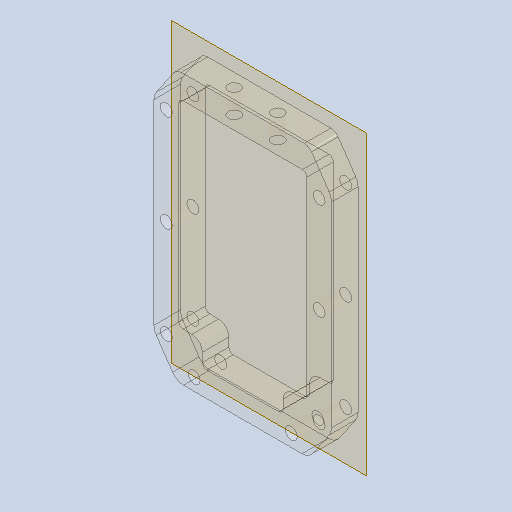
# Autodesk Inventor part: _inner
Saved by Autodesk Inventor 2024.3 (Build 283343000, 343)
## iProperties
Created: 2024-09-09
Part Number: _inner
Material: PMMA 플라스틱
Document SubType Name: Modeling
Designer: gretc
Density: 1.188 g/cm^3
Appearance: 폴리카보네이트 - 선명
Mass: 6.58685 g
Surface Area: 43.9029 cm^2
Volume: 5.54449 cm^3
Author: gretc
Autodesk Inventor part; units mm, degrees
ref_plane "YZ Plane" through (0, 0, 0) normal (1, 0, 0) x (0, 1, 0)
ref_plane "XZ Plane" through (0, 0, 0) normal (0, 1, 0) x (-1, 0, 0)
ref_plane "XY Plane" through (0, 0, 0) normal (0, 0, 1) x (1, 0, 0)
ref_plane "작업 평면1" through (0, 0, 0) normal (0, 0, 1) x (1, 0, 0)
sketch "스케치1" plane through (0, 0, 0) normal (0, 0, 1) x (1, 0, 0)
  arc A0 (-19.5808, 6.2636) -> (-20.1, 4.5766) centre (-17.1, 4.5766) ccw projected
  line L0 (-20.1, -39.6766) -> (-20.1, 4.5766) projected
  arc A1 (-20.1, -39.6766) -> (-19.5808, -41.3636) centre (-17.1, -39.6766) ccw projected
  line L1 (-15.8929, -46.7869) -> (-19.5808, -41.3636) projected
  arc A2 (-15.8929, -46.7869) -> (-13.4121, -48.1) centre (-13.4121, -45.1) ccw projected
  line L2 (13.4121, -48.1) -> (-13.4121, -48.1) projected
  arc A3 (13.4121, -48.1) -> (15.8929, -46.7869) centre (13.4121, -45.1) ccw projected
  line L3 (19.5808, -41.3636) -> (15.8929, -46.7869) projected
  arc A4 (19.5808, -41.3636) -> (20.1, -39.6766) centre (17.1, -39.6766) ccw projected
  line L4 (20.1, 4.5766) -> (20.1, -39.6766) projected
  arc A5 (20.1, 4.5766) -> (19.5808, 6.2636) centre (17.1, 4.5766) ccw projected
  line L5 (15.5953, 12.1246) -> (19.5808, 6.2636) projected
  arc A6 (15.5953, 12.1246) -> (13.9414, 13) centre (13.9414, 11) ccw projected
  line L6 (7.65, 13) -> (13.9414, 13) projected
  arc A7 (9.15, 11.5) -> (7.65, 13) centre (7.65, 11.5) ccw projected
  line L7 (9.15, 11.5) -> (9.15, 10) projected
  arc A8 (9.15, 10) -> (11.5, 7.65) centre (11.5, 10) ccw projected
  line L8 (11.5, 7.65) -> (13.5, 7.65) projected
  arc A9 (14.5, 6.65) -> (13.5, 7.65) centre (13.5, 6.65) ccw projected
  line L9 (14.5, 6.65) -> (14.5, -36.15) projected
  arc A10 (13.5, -37.15) -> (14.5, -36.15) centre (13.5, -36.15) ccw projected
  line L10 (13.5, -37.15) -> (11.5, -37.15) projected
  arc A11 (11.5, -37.15) -> (9.15, -39.5) centre (11.5, -39.5) ccw projected
  line L11 (9.15, -39.5) -> (9.15, -41.5) projected
  arc A12 (8.15, -42.5) -> (9.15, -41.5) centre (8.15, -41.5) ccw projected
  line L12 (8.15, -42.5) -> (-8.15, -42.5) projected
  arc A13 (-9.15, -41.5) -> (-8.15, -42.5) centre (-8.15, -41.5) ccw projected
  line L13 (-9.15, -41.5) -> (-9.15, -39.5) projected
  arc A14 (-9.15, -39.5) -> (-11.5, -37.15) centre (-11.5, -39.5) ccw projected
  line L14 (-11.5, -37.15) -> (-13.5, -37.15) projected
  arc A15 (-14.5, -36.15) -> (-13.5, -37.15) centre (-13.5, -36.15) ccw projected
  line L15 (-14.5, -36.15) -> (-14.5, 6.65) projected
  arc A16 (-13.5, 7.65) -> (-14.5, 6.65) centre (-13.5, 6.65) ccw projected
  line L16 (-13.5, 7.65) -> (-11.5, 7.65) projected
  arc A17 (-11.5, 7.65) -> (-9.15, 10) centre (-11.5, 10) ccw projected
  line L17 (-9.15, 10) -> (-9.15, 11.5) projected
  arc A18 (-7.65, 13) -> (-9.15, 11.5) centre (-7.65, 11.5) ccw projected
  line L18 (-13.9414, 13) -> (-7.65, 13) projected
  arc A19 (-13.9414, 13) -> (-15.5953, 12.1246) centre (-13.9414, 11) ccw projected
  line L19 (-19.5808, 6.2636) -> (-15.5953, 12.1246) projected
  circle A20 centre (17.3, 4) radius 1.35 projected
  circle A21 centre (17.3, -18) radius 1.35 projected
  circle A22 centre (11, -45.3) radius 1.35 projected
  circle A23 centre (-17.3, 4) radius 1.35 projected
  circle A24 centre (-17.3, -18) radius 1.35 projected
  circle A25 centre (-11, -45.3) radius 1.35 projected
  circle A26 centre (17.3, -40) radius 1.35 projected
  circle A27 centre (-17.3, -40) radius 1.35 projected
  line L20 (-11.5, 7.65) -> (11.5, 7.65)
  line L21 (11.5, 7.65) -> (11.5, 13)
  line L22 (11.5, 13) -> (-11.5, 13)
  line L23 (-11.5, 13) -> (-11.5, 7.65)
  point P0 (0, 0)
  constraints: 8 end point, 2 parallel, 1 horizontal, 1 perpendicular, 1 point on circle, 1 tangent
extrude "돌출1" add sketch "스케치1" along normal blind 6 contours L19 A19 L18 L23 L16 A16 L15 A15 L14 A14 L13 A13 L12 A12 L11 A11 L10 A10 L9 A9 L8 L21 L6 A6 L5 A5 L4 A4 L3 A3 L2 A2 L1 A1 L0 A0 | L18 A18 L17 A17 L23 | L22 A7 L7 A8 L20 A17 L17 A18 | L6 L21 A8 L7 A7
sketch "스케치2" plane through (-13.9414, 13, 0) normal (0, 1, 0) x (1, 0, 0)
  circle A0 centre (18.8828, -3) radius 1.35 projected
  circle A1 centre (9, -3) radius 1.35 projected
  point P0 (13.9414, 0)
extrude "돌출2" cut sketch "스케치2" against normal blind 6
